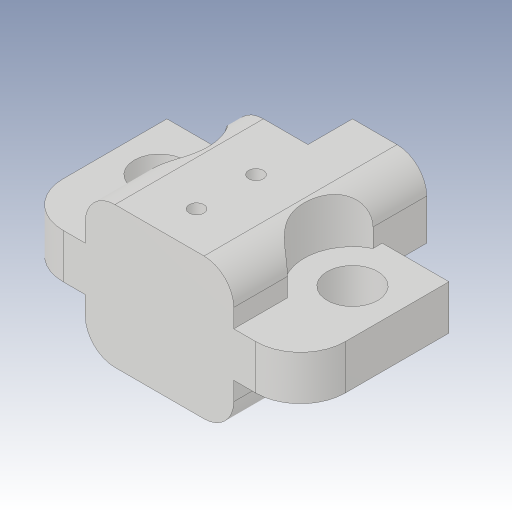
# Autodesk Inventor part: BT015_huenin20_23
Saved by Autodesk Inventor 2023.3 (Build 273359000, 359)
## iProperties
Company: HTBLA Kaindorf
RuleStatus: InUse
Created: 2024-01-24
Part Number: BT015_huenin20_23
Project: Fiberprinter-Hotend
Material: E360
Description: SMN_Gehäuse
Document SubType Name: Modeling
Designer: huenin20
Density: 7.85 g/cm^3
Appearance: Metall
Mass: 6.90708 g
Surface Area: 11.0043 cm^2
Volume: 0.879883 cm^3
AfterDocNew0: iProperties-Editor_aufrufen
Author: nicob
Keywords: 2023
Autodesk Inventor part; units mm, degrees
ref_plane "YZ Plane" through (0, 0, 0) normal (1, 0, 0) x (0, 1, 0)
ref_plane "XZ Plane" through (0, 0, 0) normal (0, 1, 0) x (-1, 0, 0)
ref_plane "XY Plane" through (0, 0, 0) normal (0, 0, 1) x (1, 0, 0)
sketch "Skizze3" plane through (0, 0, 0) normal (1, 0, 0) x (0, 1, 0)
  line L0 (3, 9.5) -> (-3, 9.5)
  line L1 (-5, 7.5) -> (-5, 2)
  line L2 (-3, 0) -> (3, 0)
  line L3 (5, 2) -> (5, 7.5)
  arc A0 (5, 7.5) -> (3, 9.5) centre (3, 7.5) ccw
  arc A1 (-3, 9.5) -> (-5, 7.5) centre (-3, 7.5) ccw
  arc A2 (-5, 2) -> (-3, 0) centre (-3, 2) ccw
  arc A3 (3, 0) -> (5, 2) centre (3, 2) ccw
  line L4 (-5, 6.25) -> (-9.5, 6.25)
  line L5 (-9.5, 6.25) -> (-9.5, 3.25)
  line L6 (-9.5, 3.25) -> (-5, 3.25)
  line L7 (5, 6.25) -> (9.5, 6.25)
  line L8 (9.5, 6.25) -> (9.5, 3.25)
  line L9 (9.5, 3.25) -> (5, 3.25)
  point P0 (-5, 0)
  point P1 (-5, 9.5)
  point P2 (5, 0)
  point P3 (0, 0)
  point P4 (0, 0)
  point P5 (-9.5, 4.75)
  point P6 (-5, 4.75)
  point P7 (9.5, 4.75)
  point P8 (5, 4.75)
  dimension "d12" = 10
  dimension "d13" = 9.5
  dimension "d14" = 2
  dimension "d83" = 4.5
  dimension "d84" = 3
  constraints: 20 end point, 10 point on line, 8 point on circle, 8 tangent, 5 midpoint, 5 perpendicular, 4 centre point, 3 equal radius, 3 horizontal, 2 equal length, 2 horizontal alignment, 2 parallel, 1 coincident
  measures "d12" distance of point (5, 0) point (-5, 0)
  measures "d13" distance of point (-5, 0) point (-5, 9.5)
  measures "d14" radius of A0
  measures "d83" distance of L4.start L4.end
  measures "d84" distance of L4.end L5.end
extrude "Extrusion3" add sketch "Skizze3" along normal blind 10 and the other way blind 3 contours A0 L3 A3 L2 A2 L1 A1 L0
extrude "Extrusion4" add sketch "Skizze3" along normal blind 10 and the other way blind 3 contours L7 L8 L9 L3 | L1 L6 L5 L4
fillet "Rundung1" radius 3 4 edges at (-3, -9.5, 4.75) (10, -9.5, 4.75) (10, 9.5, 4.75) (-3, 9.5, 4.75)
sketch "Skizze5" plane through (-3, 0, 0) normal (-1, 0, 0) x (0, 0, 1)
  line L0 (2, -5) -> (7.5, -5) projected
  line L1 (9.5, -3) -> (9.5, 3) projected
  point P0 (0, 0)
  point P1 (4.75, 0)
  point P2 (4.75, -5)
  point P3 (9.5, 0)
  constraints: 2 midpoint, 1 horizontal alignment, 1 vertical alignment
hole "Bohrung3" at (-3, 0, 4.75) direction (1, 0, 0) diameter 6 depth 12
sketch "Skizze6" plane through (-3, -3, 9.5) normal (0, 0, 1) x (1, 0, 0)
  line L0 (0, 0) -> (0, 6) projected
  point P0 (3, 3)
  point P1 (3, 3)
  point P2 (0, 3)
  point P3 (0, 3)
  dimension "d41" = 3
  constraints: 1 horizontal alignment, 3 other
  measures "d41" distance of point (0, 3) point (3, 3)
sketch "Skizze7" plane through (-3, -3, 9.5) normal (0, 0, 1) x (1, 0, 0)
  line L0 (13, 6) -> (13, 0) projected
  line L1 (0, 0) -> (0, 6) projected
  line L2 (12, 6) -> (12, 0) projected
  point P0 (6.5, 3)
  point P1 (13, 3)
  dimension "d122" = 5.5
  constraints: 1 horizontal alignment, 1 midpoint
  measures "d122" distance from line of L2 point (6.5, 3)
hole "Bohrung5" at (3.5, 0, 9.5) direction (0, 0, -1) diameter 1 end through all
sketch "Skizze9" plane through (0, -5, 6.25) normal (0, 0, 1) x (1, 0, 0)
  arc A0 (-3, -1.5) -> (0, -4.5) centre (0, -1.5) ccw projected
  line L0 (-3, 0) -> (10, 0) projected
  arc A1 (0, 14.5) -> (-3, 11.5) centre (0, 11.5) ccw projected
  line L1 (10, 10) -> (-3, 10) projected
  line L2 (-3, 10) -> (-3, 11.5) projected
  line L3 (10, 11.5) -> (10, 10) projected
  line L4 (10, 0) -> (10, -1.5) projected
  line L5 (-3, -1.5) -> (-3, 0) projected
  arc A2 (10, 11.5) -> (7, 14.5) centre (7, 11.5) ccw projected
  line L6 (7, 14.5) -> (0, 14.5) projected
  line L7 (0, -4.5) -> (7, -4.5) projected
  arc A3 (7, -4.5) -> (10, -1.5) centre (7, -1.5) ccw projected
  point P0 (0, 5)
  point P1 (3.5, -1.5)
  point P2 (3.5, 11.5)
  point P3 (3.5, 14.5)
  point P4 (3.5, -4.5)
  constraints: 3 vertical alignment, 2 horizontal alignment, 2 midpoint
hole "Bohrung6" at (3.5, 6.5, 6.25) at (3.5, -6.5, 6.25) direction (0, 0, -1) diameter 3.4 end through all start extended yes clearance for "Inbusschraube DIN EN ISO 4762" size "M3" standard "DIN"
hole "Bohrung7" at (3.5, -6.5, 6.25) at (3.5, 6.5, 6.25) direction (0, 0, 1) diameter 3.4 end through all counterbore diameter 6.5 counterbore depth 3.4 clearance for "Inbusschraube DIN EN ISO 4762" size "M3" standard "DIN"
sketch "Skizze10" plane through (10, -5, 3.25) normal (0, 0, -1) x (-1, 0, 0)
  arc A0 (5.7, 0) -> (7.3, 0) centre (6.5, -1.5) ccw projected
  arc A1 (7.3, 10) -> (5.7, 10) centre (6.5, 11.5) ccw projected
  point P0 (10, 5)
hole "Bohrung8" at (3.5, -6.5, 3.25) at (3.5, 6.5, 3.25) direction (0, 0, -1) diameter 3.4 end through all counterbore diameter 6.5 counterbore depth 3.4 clearance for "Inbusschraube DIN EN ISO 4762" size "M3" standard "DIN"
sketch "Skizze11" plane through (-3, 0, 0) normal (-1, 0, 0) x (0, 0, 1)
  circle A0 centre (4.75, 0) radius 3 projected
  line L0 (3.25, 6.5) -> (6.25, 6.5) projected
  line L1 (3.25, 6.5) -> (3.25, 5) projected
  line L2 (3.25, 5) -> (2, 5) projected
  arc A1 (2, 5) -> (0, 3) centre (2, 3) ccw projected
  line L3 (0, 3) -> (0, -3) projected
  arc A2 (0, -3) -> (2, -5) centre (2, -3) ccw projected
  line L4 (2, -5) -> (3.25, -5) projected
  line L5 (3.25, -5) -> (3.25, -6.5) projected
  line L6 (6.25, -6.5) -> (3.25, -6.5) projected
  line L7 (6.25, -6.5) -> (6.25, -5) projected
  line L8 (6.25, -5) -> (7.5, -5) projected
  arc A3 (7.5, -5) -> (9.5, -3) centre (7.5, -3) ccw projected
  line L9 (9.5, -3) -> (9.5, 3) projected
  arc A4 (9.5, 3) -> (7.5, 5) centre (7.5, 3) ccw projected
  line L10 (7.5, 5) -> (6.25, 5) projected
  line L11 (6.25, 5) -> (6.25, 6.5) projected
  line L12 (6.25, 5) -> (3.25, 5)
  line L13 (1.1282, 4.8) -> (8.3718, 4.8) projected
  line L14 (6.25, -3.25) -> (6.25, -5) projected
  line L15 (6.25, -5) -> (3.25, -5)
  line L16 (1.1282, -4.8) -> (8.3718, -4.8) projected
  line L17 (9.5, -3) -> (9.5, 3) projected
  line L18 (9.5, 0) -> (0, 0)
  line L19 (3.25, 9.5) -> (3.25, 6.5) projected
  line L20 (3.25, 6.5) -> (6.25, 6.5) projected
  line L21 (6.25, 6.5) -> (6.25, 9.5) projected
  line L22 (6.25, 9.5) -> (3.25, 9.5) projected
  line L23 (6.25, -9.5) -> (6.25, -6.5) projected
  line L24 (6.25, -6.5) -> (3.25, -6.5) projected
  line L25 (3.25, -6.5) -> (3.25, -9.5) projected
  line L26 (3.25, -9.5) -> (6.25, -9.5) projected
  line L27 (4.75, 5) -> (4.75, -5)
  point P0 (8.8514, 4.4743)
  point P1 (0.6486, -4.4743)
  point P2 (1.75, 0)
  point P3 (7.75, 0)
  point P4 (4.75, 3)
  point P5 (4.75, -3)
  constraints: 8 end point, 3 midpoint, 2 parallel, 2 point on circle, 1 perpendicular, 4 other
extrude "Extrusion7" cut sketch "Skizze11" against normal blind 3 contours L18 L27 A0 | L18 L9 A3 L16 L27 A0 | A0 L27 L18 | L27 L18 A0 | A0 L18 L3 A1 L13 L27 | A0 L18 L27 | L13 A1 L2 L12 L27 | L16 L14 L15 L27 | L12 L1 L0 L11 | L16 A3 L8 L14 | L15 L7 L6 L5 | L0 L19 L22 L21 | L23 L26 L25 L6
sketch "Skizze12" plane through (-3, 3, 9.5) normal (0, 0, 1) x (1, 0, 0)
  line L0 (12, 0) -> (12, -6) projected
  point P0 (3, -3)
  point P1 (10.5, -3)
  point P2 (12, -3)
  dimension "d113" = 1.5
  constraints: 1 horizontal alignment, 1 midpoint
  measures "d113" distance of point (12, -3) point (10.5, -3)
hole "Bohrung9" at (7.5, 0, 9.5) direction (0, 0, -1) diameter 1 depth 3.25
